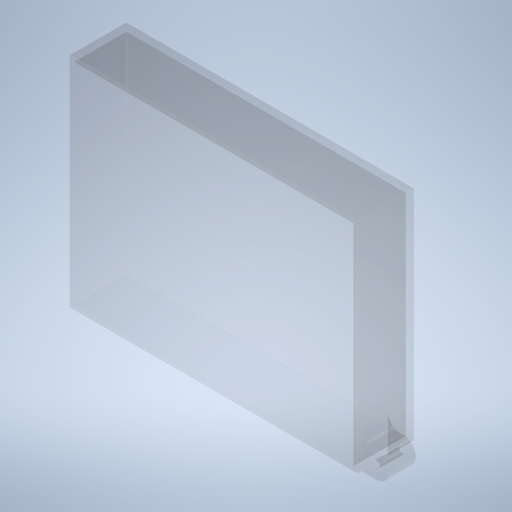
# Autodesk Inventor part: Caja de electrónica
Saved by Autodesk Inventor 2023 (Build 270158000, 158)
## iProperties
Created: 2022-03-29
Part Number: Caja de electrónica
Material: PET Plastic
Document SubType Name: Modeling
Designer: juanp
Density: 1.541 g/cm^3
Appearance: Polycarbonate - Clear
Author: juanp
Autodesk Inventor part; units mm, degrees
ref_plane "YZ Plane" through (0, 0, 0) normal (1, 0, 0) x (0, 1, 0)
ref_plane "XZ Plane" through (0, 0, 0) normal (0, 1, 0) x (-1, 0, 0)
ref_plane "XY Plane" through (0, 0, 0) normal (0, 0, 1) x (1, 0, 0)
sketch "Sketch1" plane through (0, 0, 0) normal (0, 0, 1) x (1, 0, 0)
  line L0 (0, 0) -> (280, 0)
  line L1 (394, -1) -> (3, -1)
  line L2 (3, -1) -> (3, 159)
  line L3 (3, 159) -> (394, 159)
  line L4 (394, 159) -> (394, -1)
  line L5 (0, -4) -> (397, -4)
  line L6 (397, -4) -> (397, 162)
  line L7 (397, 162) -> (0, 162)
  line L8 (0, 162) -> (0, -4)
  point P0 (280, 68.725)
  dimension "d55" = 1
  dimension "d59" = 3
  dimension "d79" = 397
  dimension "d115" = 160
  constraints: 18 end point, 4 parallel, 2 perpendicular, 1 coincident, 1 horizontal, 1 point on line, 3 other
  measures "d55" distance between parallel lines of L1 L0
  measures "d59" distance between parallel lines of L1 L5
  measures "d79" distance between parallel lines of L8 L6
  measures "d115" distance between parallel lines of L1 L3
extrude "Extrusion1" add sketch "Sketch1" against normal blind 3 contours L1 L2 L3 L4 | L8 L7 L6 L5
extrude "Extrusion2" add sketch "Sketch1" along normal blind 40
sketch "Sketch3" plane through (0, 0, 40) normal (0, 0, 1) x (1, 0, 0)
  line L0 (397, -4) -> (397, 162) projected
  line L1 (397, 162) -> (0, 162) projected
  line L2 (0, 162) -> (0, -4) projected
  line L3 (0, -4) -> (397, -4) projected
  line L4 (394, -1) -> (3, -1) projected
  line L5 (3, -1) -> (3, 159) projected
  line L6 (3, 159) -> (394, 159) projected
  line L7 (394, 159) -> (394, -1) projected
  point P0 (0, 0)
extrude "Extrusion4" add sketch "Sketch3" along normal blind 3 separate body contours L3 L2 L1 L0 | L4 L5 L6 L7
sketch "Sketch5" plane through (0, -4, -3) normal (-1, 0, 0) x (0, 0, 1)
  line L0 (0, 0) -> (20, 0) construction
  line L1 (0, 0) -> (43, 0) projected
  line L2 (20, 0) -> (20, 10) construction
  line L3 (40, 0) -> (20, 0)
  line L4 (20, 0) -> (20, 20)
  line L5 (20, 20) -> (40, 20)
  line L6 (40, 20) -> (40, 0)
  line L7 (43, 166) -> (43, 0) projected
  point P0 (3, 4)
  point P1 (20, 0)
  dimension "d84" = 20
  dimension "d85" = 10
  dimension "d106" = 20
  constraints: 12 end point, 2 parallel, 2 perpendicular, 2 point on line, 1 horizontal, 1 midpoint
  measures "d84" distance of L0.start L0.end
  measures "d85" distance of L2.end L0.end
  measures "d106" distance between parallel lines of L6 L4
extrude "Extrusion6" add sketch "Sketch5" along normal blind 21.5 bodies 1
ref_plane "Work Plane1" through (198.5, -4, -3) normal (-1, 0, 0) x (0, 0, 1)
fillet "Fillet1" radius 10 2 edges at (-21.5, 16, 27) (-21.5, -4, 27)
mirror "Mirror1" about plane through (198.5, -4, -3) normal (-1, 0, 0) of "Extrusion6", "Fillet1" bodies 1
sketch "Sketch6" plane through (0, 0, 40) normal (0, 0, 1) x (1, 0, 0)
  circle A0 centre (408.5, 6) radius 2.65
  circle A1 centre (-11.5, 6) radius 2.65
  arc A2 (408.5, -4) -> (408.5, 16) centre (408.5, 6) ccw projected
  arc A3 (-11.5, 16) -> (-11.5, -4) centre (-11.5, 6) ccw projected
  point P0 (0, 0)
  dimension "d89" = 5.3
  dimension "d90" = 5.3
  constraints: 2 centre point, 2 concentric, 1 coincident
  measures "d89" diameter of A0
  measures "d90" diameter of A1
extrude "Extrusion7" cut sketch "Sketch6" against normal through all bodies 1
fillet "Fillet2" radius 10 2 edges at (0, 16, 27) (397, 16, 27)
ref_plane "Work Plane2" through (198.5, -4, -3) normal (-1, 0, 0) x (0, 0, 1)
sketch "Sketch8" plane through (198.5, -4, -3) normal (-1, 0, 0) x (0, 0, 1)
  line L0 (-199.6845, 306.385) -> (183.5952, 306.385)
  line L1 (183.5952, 306.385) -> (183.5952, -177.7892)
  line L2 (183.5952, -177.7892) -> (-199.6845, -177.7892)
  line L3 (-199.6845, -177.7892) -> (-199.6845, 306.385)
  point P0 (3, 4)
  constraints: 8 end point, 2 parallel, 1 horizontal, 1 perpendicular
extrude "Extrusion9" cut sketch "Sketch8" along normal through all bodies 1
sketch "Sketch9" plane through (198.5, -4, -3) normal (-1, 0, 0) x (0, 0, 1)
  line L0 (3, 3) -> (43, 3) projected
  line L1 (3, 163) -> (3, 3) projected
  line L2 (43, 163) -> (3, 163) projected
  line L3 (43, 166) -> (43, 163) projected
  line L4 (0, 166) -> (43, 166) projected
  line L5 (0, 0) -> (0, 166) projected
  line L6 (43, 0) -> (0, 0) projected
  line L7 (43, 3) -> (43, 0) projected
  point P0 (3, 4)
extrude "Extrusion10" add sketch "Sketch9" along normal blind 20 bodies 1
sketch "Sketch10" plane through (178.5, -4, -3) normal (-1, 0, 0) x (0, 0, 1)
  line L0 (3, 163) -> (43, 163) projected
  line L1 (43, 163) -> (43, 166) projected
  line L2 (43, 166) -> (0, 166) projected
  line L3 (0, 166) -> (0, 0) projected
  line L4 (0, 0) -> (43, 0) projected
  line L5 (43, 0) -> (43, 3) projected
  line L6 (43, 3) -> (3, 3) projected
  line L7 (3, 3) -> (3, 163) projected
  line L8 (3, 163) -> (43, 163) projected
  line L9 (43, 163) -> (43, 3)
  line L10 (40, 0) -> (40, 30) projected
  point P0 (3, 4)
  constraints: 2 end point, 1 parallel
extrude "Extrusion11" add sketch "Sketch10" against normal blind 3 contours L0 L9 L6 L7 bodies 1
body "Solid1"
body "Solid2"
